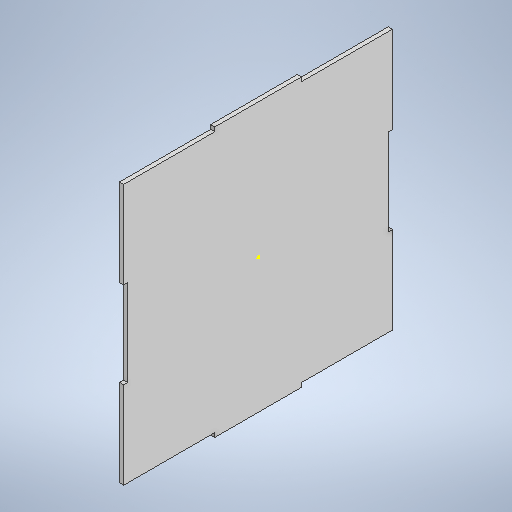
# Autodesk Inventor part: FUNDO POÇO
Saved by Autodesk Inventor 2025.2 (Build 292293000, 293)
## iProperties
Created: 2025-05-08
Part Number: FUNDO POÇO
Material: Genérico
Document SubType Name: Modeling
Designer: erick
Density: 1 g/cm^3
Appearance: Padrão
Author: erick
Autodesk Inventor part; units mm, degrees
ref_plane "YZ Plane" through (0, 0, 0) normal (1, 0, 0) x (0, 1, 0)
ref_plane "XZ Plane" through (0, 0, 0) normal (0, 1, 0) x (-1, 0, 0)
ref_plane "XY Plane" through (0, 0, 0) normal (0, 0, 1) x (1, 0, 0)
sketch "Esboço1" plane through (0, 0, 0) normal (1, 0, 0) x (0, 1, 0)
  line L0 (-129, 129) -> (129, 129)
  line L1 (129, 129) -> (129, -129)
  line L2 (129, -129) -> (-129, -129)
  line L3 (-129, -129) -> (-129, 129)
  line L4 (-129, 129) -> (129, -129) construction
  line L5 (129, 129) -> (-129, -129) construction
  point P0 (0, 0)
  dimension "d0" = 258
  dimension "d1" = 258
  constraints: 12 end point, 2 midpoint, 2 parallel, 1 horizontal, 1 perpendicular
  measures "d0" distance of L0.end L1.end
  measures "d1" distance of L1.end L2.end
extrude "Extrusão1" add sketch "Esboço1" along normal mid plane 4
sketch "Esboço2" plane through (2, 0, 0) normal (1, 0, 0) x (0, 0, -1)
  line L0 (129, 129) -> (-129, 129) projected
  line L1 (-129, 129) -> (-41.5, 129)
  line L2 (-41.5, 129) -> (-41.5, 125)
  line L3 (-41.5, 125) -> (-129, 125)
  line L4 (-129, 125) -> (-129, 129)
  line L5 (129, 129) -> (41.5, 129)
  line L6 (41.5, 129) -> (41.5, 125)
  line L7 (41.5, 125) -> (129, 125)
  line L8 (129, 125) -> (129, 129)
  line L9 (-129, 129) -> (-129, -129) projected
  line L10 (-129, -129) -> (-41.5, -129)
  line L11 (-41.5, -129) -> (-41.5, -125)
  line L12 (-41.5, -125) -> (-129, -125)
  line L13 (-129, -125) -> (-129, -129)
  line L14 (129, -129) -> (129, 129) projected
  line L15 (129, -129) -> (41.5, -129)
  line L16 (41.5, -129) -> (41.5, -125)
  line L17 (41.5, -125) -> (129, -125)
  line L18 (129, -125) -> (129, -129)
  point P0 (0, 0)
  point P1 (129, -125)
  dimension "d4" = 87.5
  dimension "d5" = 4
  dimension "d6" = 87.5
  dimension "d7" = 4
  dimension "d8" = 83
  dimension "d9" = 87.5
  dimension "d10" = 4
  dimension "d11" = 87.5
  dimension "d12" = 4
  dimension "d13" = 83
  constraints: 32 end point, 8 parallel, 4 horizontal, 4 perpendicular
  measures "d4" distance of L2.end L3.end
  measures "d5" distance of L1.end L2.end
  measures "d6" distance of L6.end L7.end
  measures "d7" distance of L5.end L6.end
  measures "d8" distance between parallel lines of L6 L2
  measures "d9" distance of L11.end L12.end
  measures "d10" distance of L10.end L11.end
  measures "d11" distance of L16.end L17.end
  measures "d12" distance of L15.end L16.end
  measures "d13" distance between parallel lines of L16 L11
extrude "Extrusão2" cut sketch "Esboço2" along normal through all both and the other way through all
sketch "Esboço3" plane through (2, 0, 0) normal (1, 0, 0) x (0, 0, -1)
  line L0 (-125, 41.5) -> (-133, 41.5)
  line L1 (-133, 41.5) -> (-133, -41.5)
  line L2 (-133, -41.5) -> (-125, -41.5)
  line L3 (-125, -41.5) -> (-125, 41.5)
  line L4 (-129, -125) -> (-129, 125) projected
  line L5 (-125, 41.5) -> (-133, -41.5) construction
  line L6 (-133, 41.5) -> (-125, -41.5) construction
  line L7 (125, -41.5) -> (133, -41.5)
  line L8 (133, -41.5) -> (133, 41.5)
  line L9 (133, 41.5) -> (125, 41.5)
  line L10 (125, 41.5) -> (125, -41.5)
  line L11 (129, 125) -> (129, -125) projected
  line L12 (125, -41.5) -> (133, 41.5) construction
  line L13 (133, -41.5) -> (125, 41.5) construction
  line L14 (-41.5, 125) -> (-129, 125) projected
  line L15 (-129, -125) -> (-41.5, -125) projected
  line L16 (129, 125) -> (41.5, 125) projected
  line L17 (41.5, -125) -> (129, -125) projected
  point P0 (0, 0)
  point P1 (-129, 0)
  point P2 (129, 0)
  dimension "d16" = 83
  dimension "d17" = 8
  dimension "d18" = 8
  dimension "d19" = 83
  dimension "d20" = 83.5
  dimension "d21" = 83.5
  dimension "d22" = 83.5
  dimension "d23" = 83.5
  constraints: 24 end point, 6 midpoint, 4 parallel, 2 horizontal, 2 perpendicular
  measures "d16" distance of L7.end L8.end
  measures "d17" distance of L8.end L9.end
  measures "d18" distance of L0.start L0.end
  measures "d19" distance of L2.end L0.start
  measures "d20" distance between parallel lines of L0 L14
  measures "d21" distance between parallel lines of L15 L2
  measures "d22" distance between parallel lines of L9 L16
  measures "d23" distance between parallel lines of L17 L7
extrude "Extrusão3" cut sketch "Esboço3" along normal through all both and the other way through all
sketch "Esboço4" plane through (2, 0, 0) normal (1, 0, 0) x (0, 0, -1)
  point P0 (0, 0)
